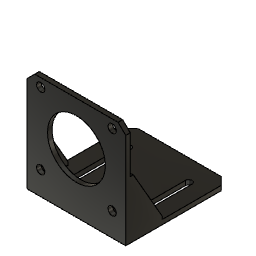
NEMA23 Motor with bracket (Autodesk Fusion 360 archive; units mm, degrees)
design "NEMA23 bracket"
Autodesk Fusion 360 part; units mm, degrees
sketch "NEMA23 bracket front" plane through (0, 0, 0) normal (0, 1, 0) x (1, 0, 0)
  line L0 (-32.5, -3) -> (-32.5, -63)
  line L1 (-32.5, 0) -> (-32.5, -3)
  line L2 (32.5, 0) -> (-32.5, 0)
  line L3 (32.5, -63) -> (32.5, -3)
  line L4 (-32.5, -3) -> (32.5, -3)
  line L5 (-27.5, -68) -> (27.5, -68)
  line L6 (23.55, -15.45) -> (-23.55, -15.45) construction
  line L7 (32.5, -3) -> (32.5, 0)
  circle A0 centre (-23.55, -62.55) radius 2.75
  line L8 (32.5, 0) -> (32.5, -68) construction
  line L9 (23.55, -62.55) -> (-23.55, -62.55) construction
  circle A1 centre (23.55, -15.45) radius 2.75
  line L10 (32.5, -3) -> (-32.5, -3)
  circle A2 centre (0, -39) radius 19.05
  line L11 (-23.55, -62.55) -> (-23.55, -15.45) construction
  line L12 (23.55, -15.45) -> (23.55, -62.55) construction
  circle A3 centre (-23.55, -15.45) radius 2.75
  circle A4 centre (23.55, -62.55) radius 2.75
  line L13 (-32.5, -63) -> (-27.5, -68)
  line L14 (27.5, -68) -> (32.5, -63)
  dimension "d22" = 38.1
  dimension "d23" = 39
  dimension "d24" = 5.5
  dimension "d27" = 47.1
  dimension "d28" = 47.1
  dimension "d29" = 47.1
  dimension "d30" = 5.5
  dimension "d31" = 5.5
  dimension "d32" = 5.5
  dimension "d33" = 68
  dimension "d34" = 32.5
  dimension "d35" = 65
  dimension "d36" = 3
  dimension "d37" = 65
  dimension "d39" = 5.45
  dimension "d46" = 5
  dimension "d47" = 5
  constraint coincident L6.start A1.centre
  constraint perpendicular L6 L12
  constraint perpendicular L9 L12
  constraint coincident L9.start L12.end
  constraint coincident A0.centre L9.end
  constraint coincident L6.end L11.end
  constraint coincident L8 L3.start
  measures "d22" diameter of A2
  measures "d23" distance of A2.centre origin
  measures "d24" diameter of A1
  measures "d27" distance of L6.end L6.start
  measures "d28" distance of L6.start L9.start
  measures "d29" distance of A0.centre L9.start
  measures "d30" diameter of A4
  measures "d31" diameter of A0
  measures "d32" diameter of A3
  measures "d33" distance of L2.start L8.end
  measures "d34" distance of L2.start origin
  measures "d35" distance of L1.start L2.start
  measures "d36" distance of L2.start L3.end
  measures "d37" distance of L3.end L0.start
  measures "d39" distance of L9.start L5
  measures "d46" distance of L8.end L5.end
  measures "d47" distance of L8.end L3.start
extrude "Extrude1" add sketch "NEMA23 bracket front" along normal blind 68 contours L1 L2 L4 L7 L10 makes body 1
extrude "Extrude2" add sketch "NEMA23 bracket front" along normal blind 3 contours L0 L3 L4 L5 L10 L13 L14 bodies 1
sketch "NEMA23 bracket side" plane through (0, 0, 0) normal (1, 0, 0) x (0, 1, 0)
  line L0 (3, 3) -> (24, 3)
  line L1 (24, 3) -> (24, 5)
  line L2 (24, 5) -> (5, 38)
  line L3 (5, 38) -> (3, 38)
  line L4 (3, 38) -> (3, 3)
  dimension "d52" = 21
  dimension "d53" = 35
  dimension "d54" = 2
  dimension "d55" = 2
  dimension "d56" = 3
  dimension "d57" = 3
  constraint horizontal L0
  constraint perpendicular L0 L1
  constraint perpendicular L1 L3
  constraint perpendicular L0 L4
  measures "d52" distance of L0.start L0.end
  measures "d53" distance of L0.start L3.end
  measures "d54" distance of L2.end L3.end
  measures "d55" distance of L0.end L1.end
  measures "d56" horizontal distance of origin L0.start
  measures "d57" vertical distance of origin L0.start
extrude "Extrude3" add sketch "NEMA23 bracket side" along normal mid plane 65 bodies 1
extrude "Extrude4" cut sketch "NEMA23 bracket side" along normal mid plane 59 bodies 1
sketch "NEMA23 bracket top" plane through (0, 0, 3) normal (0, 0, 1) x (-1, 0, 0)
  line L0 (32.5, -24) -> (29.5, -24)
  line L1 (29.5, -24) -> (29.5, -3)
  line L2 (29.5, -3) -> (-29.5, -3)
  line L3 (-29.5, -3) -> (-29.5, -24)
  line L4 (-29.5, -24) -> (-32.5, -24)
  line L5 (-32.5, -24) -> (-32.5, -68)
  line L6 (-32.5, -68) -> (32.5, -68)
  line L7 (32.5, -68) -> (32.5, -24)
  line L8 (20, -54) -> (-20, -54) construction
  line L9 (-20, -54) -> (-20, -13) construction
  line L10 (-20, -13) -> (20, -13) construction
  line L11 (20, -13) -> (20, -54) construction
  line L12 (32.5, -68) -> (27.5, -68)
  line L13 (32.5, -68) -> (32.5, -63)
  line L14 (27.5, -68) -> (32.5, -63)
  line L15 (-32.5, -68) -> (-27.5, -68)
  line L16 (-32.5, -68) -> (-32.5, -63)
  line L17 (-32.5, -63) -> (-27.5, -68)
  line L18 (22.15, -54) -> (22.15, -13)
  line L19 (17.85, -54) -> (17.85, -13)
  line L20 (-17.85, -54) -> (-17.85, -13)
  line L21 (-22.15, -54) -> (-22.15, -13)
  arc A0 (17.85, -54) -> (22.15, -54) centre (20, -54) ccw
  arc A1 (22.15, -13) -> (17.85, -13) centre (20, -13) ccw
  arc A2 (-17.85, -13) -> (-22.15, -13) centre (-20, -13) ccw
  arc A3 (-22.15, -54) -> (-17.85, -54) centre (-20, -54) ccw
  dimension "d62" = 40
  dimension "d63" = 41
  dimension "d64" = 13
  dimension "d65" = 4.3
  dimension "d66" = 4.3
  dimension "d67" = 4.3
  dimension "d68" = 4.3
  dimension "d69" = 5
  dimension "d70" = 5
  dimension "d71" = 5
  dimension "d72" = 5
  constraint horizontal L8
  constraint vertical L9
  constraint horizontal L10
  constraint vertical L11
  constraint coincident L8.start L11.end
  constraint coincident L8.end L9.start
  constraint coincident L10.end L11.start
  constraint coincident L9.end L10.start
  constraint coincident L6.end L7.start
  constraint perpendicular L7 L12
  constraint coincident L7 L13.end
  constraint coincident L5.end L6.start
  constraint coincident L6 L15.end
  constraint perpendicular L15 L16
  constraint tangent L18 A1
  constraint parallel L11 L18
  constraint coincident L8 L19.start
  constraint coincident L10 L19.end
  constraint coincident L8 L20.start
  constraint coincident L10 L20.end
  constraint tangent L21 A2
  constraint parallel L9 L21
  measures "d62" distance of L9 L11
  measures "d63" distance of L8 L10
  measures "d64" distance of origin L10
  measures "d65" diameter of A0
  measures "d66" diameter of A3
  measures "d67" diameter of A1
  measures "d68" diameter of A2
  measures "d69" distance of L6.end L12.end
  measures "d70" distance of L6.end L13.end
  measures "d71" distance of L5.end L15.end
  measures "d72" distance of L5.end L16.end
extrude "Extrude5" cut sketch "NEMA23 bracket top" against normal blind 5 contours L18 L19 A0 A1 | L20 L21 A2 A3 bodies 1
extrude "Extrude6" cut sketch "NEMA23 bracket top" against normal blind 5 contours L6 L7 L12 L13 L14 | L5 L6 L15 L16 L17 bodies 1
copy_body "Body->Comp1" bodies 1 removing the originals makes body 2 in component "NEMA23 bracket"
component "NEMA23 bracket" placed x (1, 0, 0) y (0, 1, 0) z (0, 0, 1) at (0, 0, 0)
named bodies: "NEMA23 bracket"

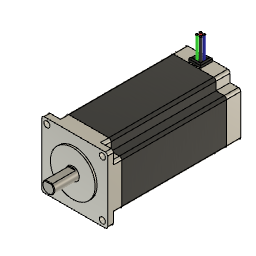
design "NEMA23 Motor 10mm shaft 113mm body"
Autodesk Fusion 360 part; units mm, degrees
sketch "Motor Front" plane through (0, 0, 0) normal (0, 1, 0) x (1, 0, 0)
  circle A0 centre (0, 0) radius 19
  line L0 (28, 28) -> (-28, 28)
  line L1 (-28, 28) -> (-28, -28)
  line L2 (-28, -28) -> (28, -28)
  line L3 (28, -28) -> (28, 28)
  line L4 (28, 28) -> (-28, -28) construction
  line L5 (-28, 28) -> (28, -28) construction
  line L6 (23.55, -23.55) -> (-23.55, -23.55) construction
  line L7 (-23.55, -23.55) -> (-23.55, 23.55) construction
  line L8 (-23.55, 23.55) -> (23.55, 23.55) construction
  line L9 (23.55, 23.55) -> (23.55, -23.55) construction
  line L10 (23.55, -23.55) -> (-23.55, 23.55) construction
  line L11 (-23.55, -23.55) -> (23.55, 23.55) construction
  circle A1 centre (-23.55, -23.55) radius 2.55
  circle A2 centre (23.55, -23.55) radius 2.55
  circle A3 centre (-23.55, 23.55) radius 2.55
  circle A4 centre (23.55, 23.55) radius 2.55
  line L12 (-28, -28) -> (-19, -28)
  line L13 (-19, -28) -> (-19, -19)
  line L14 (-19, -19) -> (-28, -19)
  line L15 (-28, -19) -> (-28, -28)
  line L16 (28, -28) -> (19, -28)
  line L17 (19, -28) -> (19, -19)
  line L18 (19, -19) -> (28, -19)
  line L19 (28, -19) -> (28, -28)
  line L20 (28, 28) -> (19, 28)
  line L21 (19, 28) -> (19, 19)
  line L22 (19, 19) -> (28, 19)
  line L23 (28, 19) -> (28, 28)
  line L24 (-28, 28) -> (-19, 28)
  line L25 (-19, 28) -> (-19, 19)
  line L26 (-19, 19) -> (-28, 19)
  line L27 (-28, 19) -> (-28, 28)
  circle A5 centre (0, 0) radius 5.5
  dimension "d1" = 38
  dimension "d2" = 56
  dimension "d3" = 56
  dimension "d4" = 47.1
  dimension "d5" = 47.1
  dimension "d6" = 5.1
  dimension "d7" = 5.1
  dimension "d8" = 5.1
  dimension "d9" = 5.1
  dimension "d10" = 9
  dimension "d11" = 9
  dimension "d12" = 9
  dimension "d13" = 9
  dimension "d14" = 9
  dimension "d15" = 9
  dimension "d16" = 9
  dimension "d17" = 9
  dimension "d20" = 11
  constraint coincident A0.centre A5.centre
  constraint perpendicular L0 L1
  constraint parallel L0 L2
  constraint parallel L1 L3
  constraint horizontal L0
  constraint coincident L4 A0.centre
  constraint coincident L5 A0.centre
  constraint perpendicular L6 L7
  constraint parallel L6 L8
  constraint parallel L7 L9
  constraint horizontal L6
  constraint coincident L10 A0.centre
  constraint coincident L11 A0.centre
  constraint coincident L6.end L7.start
  constraint coincident L6.start L9.end
  constraint coincident L7.end L8.start
  constraint coincident L8.end L9.start
  constraint horizontal L12
  constraint vertical L13
  constraint horizontal L14
  constraint vertical L15
  constraint horizontal L16
  constraint vertical L17
  constraint horizontal L18
  constraint vertical L19
  constraint horizontal L20
  constraint vertical L21
  constraint horizontal L22
  constraint vertical L23
  constraint horizontal L24
  constraint vertical L25
  constraint horizontal L26
  constraint vertical L27
  measures "d1" diameter of A0
  measures "d2" distance of L1.end L2.end
  measures "d3" distance of L0.end L1.end
  measures "d4" distance of L7.end L8.end
  measures "d5" distance of L6.end L7.end
  measures "d6" diameter of A1 A0.centre
  measures "d7" diameter of A2 A0.centre
  measures "d8" diameter of A3
  measures "d9" diameter of A4
  measures "d10" distance of L1.end L12.end
  measures "d11" distance of L1.end L14.end
  measures "d12" distance of L2.end L16.end
  measures "d13" distance of L2.end L18.end
  measures "d14" distance of L0.start L20.end
  measures "d15" distance of L0.start L22.end
  measures "d16" distance of L0.end L24.end
  measures "d17" distance of L0.end L26.end
  measures "d20" diameter of A5
extrude "Extrude1" add sketch "Motor Front" along normal blind 5 contours A0 | L0 L3 L20 L21 L22 L23 | L0 L1 L2 L3 L13 L14 L17 L18 L21 L22 L25 L26 | L0 L1 L24 L25 L26 L27 | L2 L3 L16 L17 L18 L19 | L1 L2 L12 L13 L14 L15 | A5 makes body 1
extrude "Extrude2" cut sketch "Motor Front" along normal blind 5 contours A5 bodies 1
extrude "Extrude3" add sketch "Motor Front" along normal blind 12 contours A0 | L0 L1 L2 L3 L13 L14 L17 L18 L21 L22 L25 L26 bodies 1
extrude "Extrude4" add sketch "Motor Front" against normal blind 1.6 contours A0 bodies 1
fillet "Fillet1" radius 2 4 edges at (28, 2.5, 28) (-28, 2.5, 28) (28, 2.5, -28) (-28, 2.5, -28) on bodies 1
fillet "Fillet2" radius 2 4 edges at (28, 8.5, 19) (19, 8.5, 28) (28, 8.5, -19) (19, 8.5, -28) on bodies 1
fillet "Fillet3" radius 2 4 edges at (-19, 8.5, 28) (-28, 8.5, 19) (-28, 8.5, -19) (-19, 8.5, -28) on bodies 1
sketch "Motor Middle" plane through (0, 12, 0) normal (0, 1, 0) x (-1, 0, 0)
  circle A0 centre (0, 0) radius 5.5
  arc A1 (17, -28) -> (19, -26) centre (17, -26) ccw
  line L0 (19, -26) -> (19, -19)
  line L1 (19, -19) -> (26, -19)
  arc A2 (26, -19) -> (28, -17) centre (26, -17) ccw
  line L2 (28, -17) -> (28, 17)
  arc A3 (28, 17) -> (26, 19) centre (26, 17) ccw
  line L3 (26, 19) -> (19, 19)
  line L4 (19, 19) -> (19, 26)
  arc A4 (19, 26) -> (17, 28) centre (17, 26) ccw
  line L5 (17, 28) -> (-17, 28)
  arc A5 (-17, 28) -> (-19, 26) centre (-17, 26) ccw
  line L6 (-19, 26) -> (-19, 19)
  line L7 (-19, 19) -> (-26, 19)
  arc A6 (-26, 19) -> (-28, 17) centre (-26, 17) ccw
  line L8 (-28, 17) -> (-28, -17)
  arc A7 (-28, -17) -> (-26, -19) centre (-26, -17) ccw
  line L9 (-26, -19) -> (-19, -19)
  line L10 (-19, -19) -> (-19, -26)
  arc A8 (-19, -26) -> (-17, -28) centre (-17, -26) ccw
  line L11 (-17, -28) -> (17, -28)
  line L12 (28, 28) -> (-28, 28)
  line L13 (-28, 28) -> (-28, -28)
  line L14 (-28, -28) -> (28, -28)
  line L15 (28, -28) -> (28, 28)
  line L16 (28, 28) -> (-28, -28) construction
  line L17 (-28, 28) -> (28, -28) construction
  line L18 (28, 28) -> (19, 28)
  line L19 (19, 28) -> (19, 19)
  line L20 (19, 19) -> (28, 19)
  line L21 (28, 19) -> (28, 28)
  line L22 (-28, 28) -> (-19, 28)
  line L23 (-19, 28) -> (-19, 19)
  line L24 (-19, 19) -> (-28, 19)
  line L25 (-28, 19) -> (-28, 28)
  line L26 (28, -28) -> (19, -28)
  line L27 (19, -28) -> (19, -19)
  line L28 (19, -19) -> (28, -19)
  line L29 (28, -19) -> (28, -28)
  line L30 (-28, -28) -> (-19, -28)
  line L31 (-19, -28) -> (-19, -19)
  line L32 (-19, -19) -> (-28, -19)
  line L33 (-28, -19) -> (-28, -28)
  dimension "d30" = 56
  dimension "d31" = 56
  dimension "d32" = 9
  dimension "d33" = 9
  dimension "d34" = 9
  dimension "d35" = 9
  dimension "d36" = 9
  dimension "d37" = 9
  dimension "d38" = 9
  dimension "d39" = 9
  constraint perpendicular L12 L13
  constraint parallel L12 L14
  constraint parallel L13 L15
  constraint horizontal L12
  constraint coincident L16 A0.centre
  constraint coincident L17 A0.centre
  constraint coincident A0.centre origin
  constraint horizontal L18
  constraint vertical L19
  constraint horizontal L20
  constraint vertical L21
  constraint horizontal L22
  constraint vertical L23
  constraint horizontal L24
  constraint vertical L25
  constraint horizontal L26
  constraint vertical L27
  constraint horizontal L28
  constraint vertical L29
  constraint horizontal L30
  constraint vertical L31
  constraint horizontal L32
  constraint vertical L33
  measures "d30" distance of L13.end L14.end
  measures "d31" distance of L12.end L13.end
  measures "d32" distance of L12.start L18.end
  measures "d33" distance of L12.start L20.end
  measures "d34" distance of L12.end L22.end
  measures "d35" distance of L12.end L24.end
  measures "d36" distance of L14.end L26.end
  measures "d37" distance of L14.end L28.end
  measures "d38" distance of L13.end L30.end
  measures "d39" distance of L13.end L32.end
extrude "Extrude5" add sketch "Motor Middle" along normal blind 89 separate body contours A0 | A1 L0 L1 A2 L2 A3 L3 L4 A4 L5 A5 L6 L7 A6 L8 A7 L9 L10 A8 L11 L12 L13 L14 L15 L19 L20 L23 L24 L27 L28 L31 L32 makes body 2
extrude "Extrude6" add 1 faces at (-6.3333, 101, -6.3333) along direction (0, 1, 0) blind 12 separate body on bodies 2 makes body 3
sketch "Wires" plane through (0, 0, 28) normal (0, 0, 1) x (-1, 0, 0)
  line L0 (17, -101) -> (-17, -101)
  line L1 (-17, -101) -> (-17, -113)
  line L2 (-17, -113) -> (17, -113)
  line L3 (17, -113) -> (17, -101)
  line L4 (5, -102) -> (-5, -102)
  line L5 (-5, -102) -> (-5, -112)
  line L6 (-5, -112) -> (5, -112)
  line L7 (5, -112) -> (5, -102)
  line L8 (3, -110) -> (-3, -110)
  line L9 (-3, -110) -> (-3, -104)
  line L10 (-3, -104) -> (3, -104)
  line L11 (3, -104) -> (3, -110)
  line L12 (1.5, -108.5) -> (-1.5, -108.5) construction
  line L13 (-1.5, -108.5) -> (-1.5, -105.5) construction
  line L14 (-1.5, -105.5) -> (1.5, -105.5) construction
  line L15 (1.5, -105.5) -> (1.5, -108.5) construction
  circle A0 centre (1.5, -108.5) radius 0.75
  circle A1 centre (-1.5, -108.5) radius 0.75
  circle A2 centre (1.5, -105.5) radius 0.75
  circle A3 centre (-1.5, -105.5) radius 0.75
  circle A4 centre (1.5, -108.5) radius 1
  circle A5 centre (-1.5, -108.5) radius 1
  circle A6 centre (1.5, -105.5) radius 1
  circle A7 centre (-1.5, -105.5) radius 1
  dimension "d90" = 1.5
  dimension "d91" = 1.5
  dimension "d92" = 1.5
  dimension "d93" = 1.5
  constraint horizontal L4
  constraint vertical L5
  constraint horizontal L6
  constraint vertical L7
  constraint horizontal L8
  constraint vertical L9
  constraint horizontal L10
  constraint vertical L11
  constraint horizontal L12
  constraint vertical L13
  constraint horizontal L14
  constraint vertical L15
  constraint coincident L12.start L15.end
  constraint coincident L12.end L13.start
  constraint coincident L14.end L15.start
  constraint coincident L13.end L14.start
  constraint concentric A0 A4
  constraint concentric A1 A5
  constraint concentric A2 A6
  constraint concentric A3 A7
  measures "d90" diameter of A0
  measures "d91" diameter of A1
  measures "d92" diameter of A2
  measures "d93" diameter of A3
sketch "Shaft" plane through (0, 0, 0) normal (0, 1, 0) x (1, 0, 0)
  circle A0 centre (0, 0) radius 5
  line L0 (3, -4) -> (-3, -4)
  dimension "d62" = 10
  dimension "d63" = 4
  constraint coincident A0.centre origin
  constraint horizontal L0
  constraint coincident A0 L0.end
  constraint coincident A0 L0.start
  measures "d62" diameter of A0
  measures "d63" distance of L0 A0.centre
extrude "Extrude10" add sketch "Shaft" along normal blind 12 separate body makes body 4
extrude "Extrude11" add sketch "Shaft" 1 faces at (1.0842, 0, 2.1187) along normal blind 2.4 contours A0 L0 picked at (0.7998, -4.1289) on bodies 4 bodies 4
extrude "Extrude12" add sketch "Shaft" against normal blind 22.4 contours A0 L0 picked at (1.1226, 0.6118) bodies 4
extrude "Extrude13" add sketch "Shaft" against normal blind 2.4 contours A0 L0 picked at (0.7998, -4.1289) bodies 4
chamfer "Chamfer1" distance 0.5 angle 45 2 edges at (0, -22.4, 4) (0, -22.4, -5) on bodies 4
copy_body "CutPasteBodies1" bodies 1 2 3 removing the originals makes body 5 makes body 6 makes body 7 in component "Body"
copy_body "Body->Comp1" bodies 4 removing the originals makes body 8 in component "Shaft"
extrude "Extrude1'" add sketch "Wires" along normal blind 19.99 contours A0 | A1 | A2 | A3 bodies 7 in component "Body"
extrude "Extrude2'" add sketch "Wires" along normal blind 20 contours A4 | A5 | A6 | A7 bodies 7 in component "Body"
extrude "Extrude3'" add sketch "Wires" along normal blind 3 contours L4 L5 L6 L7 bodies 7 in component "Body"
fillet "Fillet1'" radius 1 8 edges at (-5, 107, 31) (0, 112, 31) (0, 102, 31) (5, 107, 31) (3, 107, 31) (0, 110, 31) (-3, 107, 31) (0, 104, 31) on bodies 7 in component "Body"
extrude "Extrude4'" add sketch "Wires" along normal blind 0.5 contours L8 L9 L10 L11 bodies 7 in component "Body"
component "Motor" placed x (1, 0, 0) y (0, 1, 0) z (0, 0, 1) at (0, 0, 0)
component "Body" placed x (1, 0, 0) y (0, 1, 0) z (0, 0, 1) at (0, 0, 0) in component "Motor"
component "Shaft" placed x (1, 0, 0) y (0, 1, 0) z (0, 0, 1) at (0, 0, 0) in component "Motor"
named bodies: "Front", "Middle", "Back", "Shaft", "Back (1)"
